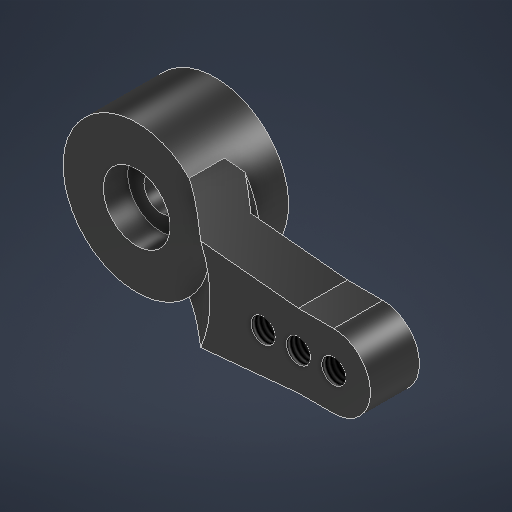
# Autodesk Inventor part: ARRMA_1_7_25t_servo_arm
Saved by Autodesk Inventor 2026 (Build 300175000, 175)
## iProperties
Created: 2025-08-23
Part Number: ARRMA_1_7_25t_servo_arm
Material: Aluminum 6061
Document SubType Name: Modeling
Designer: gisen
Density: 2.7 g/cm^3
Appearance: Glossy - Black
Author: gisen
Autodesk Inventor part; units mm, degrees
ref_plane "YZ Plane" through (0, 0, 0) normal (1, 0, 0) x (0, 1, 0)
ref_plane "XZ Plane" through (0, 0, 0) normal (0, 1, 0) x (-1, 0, 0)
ref_plane "XY Plane" through (0, 0, 0) normal (0, 0, 1) x (1, 0, 0)
sketch "Sketch1" plane through (0, 0, 0) normal (0, 0, 1) x (1, 0, 0)
  circle A0 centre (0, 0) radius 7.5
  line L0 (24.5, 0) -> (17.3, 0) construction
  line L1 (24.5, 3.75) -> (17.3, 3.75)
  line L2 (17.3, -3.75) -> (24.5, -3.75)
  arc A1 (24.5, -3.75) -> (24.5, 3.75) centre (24.5, 0) ccw
  arc A2 (17.3, 3.75) -> (17.3, -3.75) centre (17.3, 0) ccw
  line L3 (20.9, 3.75) -> (5.3561, 5.25)
  line L4 (20.9, -3.75) -> (5.3561, -5.25)
  point P0 (20.9, 0)
  dimension "d0" = 15
  dimension "d2" = 7.5
  dimension "d5" = 24.5
  dimension "d6" = 10.5
  dimension "d52" = 17.3
  constraints: 12 end point, 6 point on circle, 4 tangent, 3 centre point, 3 midpoint, 1 coincident, 1 horizontal, 1 parallel, 1 point on line, 1 vertical alignment
  measures "d0" diameter of A0
  measures "d2" diameter of A2
  measures "d5" distance of L0.start point (0, 0)
  measures "d6" distance of L4.end L3.end
  measures "d52" distance of L0.end point (0, 0)
extrude "Extrusion1" add sketch "Sketch1" along normal blind 12.4
sketch "Sketch3" plane through (0, 0, 12.4) normal (0, 0, 1) x (1, 0, 0)
  arc A0 (5.3561, 5.25) -> (5.3561, -5.25) centre (0, 0) ccw projected
  circle A1 centre (0, 0) radius 7.5
  point P0 (5.3561, 5.25)
  constraints: 1 coincident, 3 other
extrude "Extrusion2" cut sketch "Sketch3" against normal blind 4.4
sketch "Sketch6" plane through (0, 0, 8) normal (0, 0, 1) x (1, 0, 0)
  point P0 (0, 0)
hole "Hole2" at (0, 0, 8) direction (0, 0, -1) diameter 3.5 end through all counterbore diameter 6.8 counterbore depth 2.5
sketch "Sketch8" plane through (0, 0, 0) normal (0, 0, -1) x (-1, 0, 0)
  circle A0 centre (0, 0) radius 2.6
  dimension "d40" = 5.2
  constraints: 1 centre point, 1 coincident
  measures "d40" diameter of A0
extrude "serration" cut sketch "Sketch8" against normal blind 3.6
sketch "Sketch4" plane through (0, 0, 0) normal (0, 0, -1) x (-1, 0, 0)
  circle A0 centre (0, 0) radius 12
  arc A1 (-5.3561, -5.25) -> (-5.3561, 5.25) centre (0, 0) ccw projected
  line L0 (-20.9, 3.75) -> (-5.3561, 5.25) projected
  line L1 (-24.5, 3.75) -> (-20.9, 3.75) projected
  arc A2 (-24.5, 3.75) -> (-24.5, -3.75) centre (-24.5, 0) ccw projected
  line L2 (-20.9, -3.75) -> (-24.5, -3.75) projected
  line L3 (-5.3561, -5.25) -> (-20.9, -3.75) projected
  point P0 (-11.0407, -4.7014)
  point P1 (-11.0407, 4.7014)
  dimension "d13" = 24
  constraints: 1 centre point, 1 coincident
  measures "d13" diameter of A0
extrude "Extrusion3" cut sketch "Sketch4" against normal blind 7.4 contours A0 L3 L2 A2 L1 L0
sketch "Sketch7" plane through (0, 0, 12.4) normal (0, 0, 1) x (1, 0, 0)
  arc A0 (24.5, -3.75) -> (24.5, 3.75) centre (24.5, 0) ccw construction
  line L0 (24.5, 0) -> (17.3, 0) construction
  line L1 (24.5, -3.75) -> (17.3, -3.75)
  line L2 (17.3, 3.75) -> (24.5, 3.75)
  arc A1 (24.5, -3.75) -> (24.5, 3.75) centre (24.5, 0) ccw
  arc A2 (17.3, 3.75) -> (17.3, -3.75) centre (17.3, 0) ccw
  point P0 (0, 0)
  point P1 (20.9, 0)
  dimension "d30" = 7.2
  dimension "d32" = 7.5
  constraints: 8 end point, 4 point on circle, 4 tangent, 2 centre point, 1 horizontal, 1 midpoint, 1 parallel
  measures "d30" distance of L0.start L0.end
  measures "d32" distance between parallel lines of L1 L2
hole "Hole3" at (24.5, 0, 12.4) at (20.9, 0, 12.4) at (17.3, 0, 12.4) direction (0, 0, -1) diameter 2.459 end through all thread size "M3x0.5" class "6H" standard "ISO Metric profile"
sketch "Sketch9" plane through (0, 0, 0) normal (0, 0, -1) x (-1, 0, 0)
  arc A0 (-5.3561, -5.25) -> (-5.3561, 5.25) centre (0, 0) ccw projected
  circle A1 centre (0, 0) radius 9
  circle A2 centre (0, 0) radius 2.6 projected
  circle A3 centre (0, 0) radius 7.5
  line L0 (-11.0407, 4.7014) -> (-5.3561, 5.25) projected
  arc A4 (-11.0407, 4.7014) -> (-11.0407, -4.7014) centre (0, 0) ccw projected
  line L1 (-5.3561, -5.25) -> (-11.0407, -4.7014) projected
  point P0 (-5.3561, -5.25)
  dimension "d43" = 1.5
  constraints: 2 coincident, 1 centre point, 3 other
  measures "d43" radial gap between concentric circles of A0 A1
extrude "Extrusion5" cut sketch "Sketch9" against normal blind 4.4 contours L1 A1 L0 A3 | L1 A4 L0 A1
chamfer "Chamfer1" distance 3 angle 45 1 edges at (12, 0, 4.4) measured on face at (11.5, 0, 4.4)
chamfer "Chamfer2" distance 4.4 angle 45 1 edges at (7.5, 0, 12.4) measured on face at (7.5, 0, 11.9)
equation "\"d30\" = d3"
equation "\"d32\" = d2"
equation "\"d3\" = 7.2"
body "Solid1"
